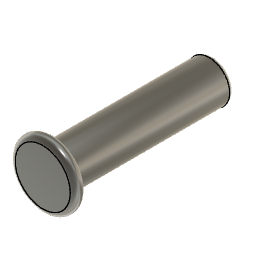
table_lamp (Autodesk Fusion 360 archive; units mm, degrees)
design "pin"
Autodesk Fusion 360 part; units mm, degrees
sketch "Sketch1" plane through (0, 0, 0) normal (0, 1, 0) x (1, 0, 0)
  circle A0 centre (0, 0) radius 7.5
  circle A1 centre (0, 0) radius 12
  dimension "d1" = 15
  dimension "d2" = 24
  constraint coincident A0.centre A1.centre
  constraint concentric A0 A1
  measures "d1" diameter of A0
  measures "d2" diameter of A1
extrude "Extrude1" add sketch "Sketch1" along normal mid plane 58 contours A0 makes body 1
extrude "Extrude2" add sketch "Sketch1" along normal blind 0 and the other way blind 4 from surface at -29 contours A0 | A1 bodies 1
fillet "Fillet1" radius 2 2 edges at (-11.1879, -33, -4.3394) (-11.1879, -29, 4.3394) on bodies 1
copy_body "Body->Comp1" bodies 1 removing the originals makes body 2 in component "Component"
fillet "Fillet1'" radius 1.5 1 edges at (-6.9925, 29, 2.7121) on bodies 2 in component "Component"
component "Component" placed x (1, 0, 0) y (0, 1, 0) z (0, 0, 1) at (0, 0, 0)
